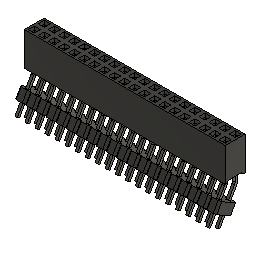
4862 CyberDeck Bonnet (Autodesk Fusion 360 archive; units mm, degrees)
design "2x20 Header 150 degree"
Autodesk Fusion 360 part; units mm, degrees
sketch "Sketch1" plane through (0, 0, 0) normal (1, 0, 0) x (0, 1, 0) in component "header"
  line L0 (-2, 0) -> (-1.7113, 0.5)
  line L1 (-1.7113, 0.5) -> (1.7113, 0.5)
  line L2 (1.7113, 0.5) -> (2, 0)
  line L3 (2, 0) -> (2.5, 0)
  line L4 (2.5, 0) -> (2.5, 8.5)
  line L5 (2.5, 8.5) -> (-2.5, 8.5)
  line L6 (-2.5, 8.5) -> (-2.5, 0)
  line L7 (-2.5, 0) -> (-2, 0)
  line L8 (0, 0.5) -> (0, 0) construction
  line L9 (0, 0.5) -> (0, 8.5) construction
  line L10 (1.27, 0.5) -> (1.27, -2.06)
  line L11 (1.27, -2.06) -> (-3.23, -9.8542)
  line L12 (-1.27, 0.5) -> (-1.27, -1)
  line L13 (-1.27, -1) -> (-5.594, -8.4894)
  line L14 (-5.594, -8.4894) -> (-3.23, -9.8542) construction
  line L15 (-5.0771, -5.3237) -> (-0.7469, -7.8237)
  line L16 (-0.7469, -7.8237) -> (0.5231, -5.624)
  line L17 (0.5231, -5.624) -> (-3.8071, -3.124)
  line L18 (-3.8071, -3.124) -> (-5.0771, -5.3237)
  line L19 (-2.912, -6.5737) -> (-4.412, -9.1718) construction
  dimension "d1" = 5
  dimension "d2" = 8.5
  dimension "d3" = 0.5
  dimension "d4" = 0.5
  dimension "d5" = 0.5
  dimension "d6" = 120
  dimension "d7" = 0.5
  dimension "d8" = 2.56
  dimension "d9" = 9
  dimension "d10" = 1.27
  dimension "d11" = 1.5
  dimension "d12" = 1.27
  dimension "d13" = 150
  dimension "d14" = 2.54
  dimension "d15" = 3
  dimension "d16" = 5
  constraint horizontal L1
  constraint parallel L1 L3
  constraint perpendicular L3 L4
  constraint perpendicular L4 L5
  constraint perpendicular L5 L6
  constraint perpendicular L6 L7
  constraint midpoint L1 L8.start
  constraint coincident L8.end origin
  constraint vertical L8
  constraint midpoint L5 L9.end
  constraint vertical L9
  constraint collinear L3 L7
  constraint coincident L1 L10.start
  constraint perpendicular L1 L10
  constraint coincident L1 L12.start
  constraint perpendicular L1 L12
  constraint parallel L11 L13
  constraint perpendicular L13 L14
  constraint coincident L11.end L14.end
  constraint perpendicular L11 L15
  constraint perpendicular L15 L16
  constraint perpendicular L17 L18
  constraint perpendicular L16 L17
  constraint coincident L15.start L18.end
  constraint midpoint L15 L19.start
  constraint midpoint L14 L19.end
  constraint perpendicular L15 L19
  measures "d1" distance of L4.end L5.end
  measures "d2" distance of L8.end L5
  measures "d3" distance of L2.end L3.end
  measures "d4" distance of L0.start L6.end
  measures "d5" distance of L1 L7
  measures "d6" angle of L0 L7
  measures "d7" distance of L8.start L8.end
  measures "d8" distance of L10.start L10.end
  measures "d9" distance of L10.end L11.end
  measures "d10" distance of L8.end L10
  measures "d11" distance of L12.start L12.end
  measures "d12" distance of L9 L12
  measures "d13" angle of L12 L13
  measures "d14" distance of L17.end L15.start
  measures "d15" distance of L19.start L19.end
  measures "d16" distance of L16.end L17.end
sketch "Sketch2" plane through (0, 0, 0) normal (0, 0, 1) x (1, 0, 0) in component "header"
  line L0 (0.95, 1.59) -> (1.59, 1.59)
  line L1 (1.59, 1.59) -> (1.59, 0.95)
  line L2 (1.59, 0.95) -> (0.95, 0.95)
  line L3 (0.95, 0.95) -> (0.95, 1.59)
  line L4 (1.27, 1.59) -> (1.27, 1.27) construction
  line L5 (1.27, 1.27) -> (1.59, 1.27) construction
  line L6 (0, 0) -> (3, 0) construction
  line L7 (0.95, -1.59) -> (1.59, -1.59)
  line L8 (1.59, -1.59) -> (1.59, -0.95)
  line L9 (1.59, -0.95) -> (0.95, -0.95)
  line L10 (0.95, -0.95) -> (0.95, -1.59)
  dimension "d19" = 0.64
  dimension "d20" = 0.64
  dimension "d21" = 1.27
  dimension "d22" = 1.27
  dimension "d45" = 3
  constraint horizontal L0
  constraint vertical L1
  constraint horizontal L2
  constraint vertical L3
  constraint midpoint L0 L4.start
  constraint perpendicular L0 L4
  constraint perpendicular L4 L5
  constraint midpoint L1 L5.end
  constraint coincident L6.start origin
  constraint horizontal L6
  constraint symmetric L0.start L6 L7.start
  constraint symmetric L0.end L6 L7.end
  constraint symmetric L1.end L6 L8.end
  constraint symmetric L2.end L6 L9.end
  measures "d19" distance of L0.start L0.end
  measures "d20" distance of L0.start L2.end
  measures "d21" distance of L5 L6.start
  measures "d22" distance of L6.start L4
  measures "d45" distance of L6.start L6.end
extrude "Extrude1" add sketch "Sketch1" along normal blind 50.8 contours L0 L1 L2 L3 L4 L5 L6 L7 makes body 1 in component "Header Female"
sweep "Sweep1" add profiles "Sketch2" path "Sketch1" along L10 L11 section 1 contours L0 L1 L2 L3 separate body makes body 2 in component "Pins"
fillet "Fillet1" radius 1 1 edges at (1.27, 0.95, -1.9743) on bodies 2 in component "Pins"
fillet "Fillet1" radius 1.5 1 edges at (1.27, 1.59, -2.1457) on bodies 2 in component "Pins"
pattern_linear "R-Pattern1" count 20 spacing 2.54 along (1, 0, 0) of bodies 2 makes body 3 at (3.49, -0.2493, -4.9048) makes body 4 at (6.03, -0.2493, -4.9048) makes body 5 at (8.57, -0.2493, -4.9048) makes body 6 at (11.11, -0.2493, -4.9048) makes body 7 at (13.65, -0.2493, -4.9048) makes body 8 at (16.19, -0.2493, -4.9048) makes body 9 at (18.73, -0.2493, -4.9048) makes body 10 at (21.27, -0.2493, -4.9048) makes body 11 at (23.81, -0.2493, -4.9048) makes body 12 at (26.35, -0.2493, -4.9048) makes body 13 at (28.89, -0.2493, -4.9048) makes body 14 at (31.43, -0.2493, -4.9048) makes body 15 at (33.97, -0.2493, -4.9048) makes body 16 at (36.51, -0.2493, -4.9048) makes body 17 at (39.05, -0.2493, -4.9048) makes body 18 at (41.59, -0.2493, -4.9048) makes body 19 at (44.13, -0.2493, -4.9048) makes body 20 at (46.67, -0.2493, -4.9048) makes body 21 at (49.21, -0.2493, -4.9048) in component "Pins"
sweep "Sweep2" add profiles "Sketch2" path "Sketch1" along L12 L13 section 1 contours L7 L8 L9 L10 separate body makes body 22 in component "Pins"
fillet "Fillet2" radius 1 1 edges at (1.27, -1.59, -0.9143) on bodies 22 in component "Pins"
fillet "Fillet2" radius 1.5 1 edges at (1.27, -0.95, -1.0857) on bodies 22 in component "Pins"
pattern_linear "R-Pattern2" count 20 spacing 2.54 along (1, 0, 0) of bodies 22 makes body 23 at (3.49, -2.7306, -3.7432) makes body 24 at (6.03, -2.7306, -3.7432) makes body 25 at (8.57, -2.7306, -3.7432) makes body 26 at (11.11, -2.7306, -3.7432) makes body 27 at (13.65, -2.7306, -3.7432) makes body 28 at (16.19, -2.7306, -3.7432) makes body 29 at (18.73, -2.7306, -3.7432) makes body 30 at (21.27, -2.7306, -3.7432) makes body 31 at (23.81, -2.7306, -3.7432) makes body 32 at (26.35, -2.7306, -3.7432) makes body 33 at (28.89, -2.7306, -3.7432) makes body 34 at (31.43, -2.7306, -3.7432) makes body 35 at (33.97, -2.7306, -3.7432) makes body 36 at (36.51, -2.7306, -3.7432) makes body 37 at (39.05, -2.7306, -3.7432) makes body 38 at (41.59, -2.7306, -3.7432) makes body 39 at (44.13, -2.7306, -3.7432) makes body 40 at (46.67, -2.7306, -3.7432) makes body 41 at (49.21, -2.7306, -3.7432) in component "Pins"
extrude "Extrude2" cut sketch "Sketch2" against normal blind 2.54 from surface at 8.5 bodies 1 in component "Header Female"
chamfer "Chamfer2" distance 0.448 angle 45 8 edges at (1.27, -0.95, 8.5) (0.95, -1.27, 8.5) (1.27, -1.59, 8.5) (1.59, -1.27, 8.5) (0.95, 1.27, 8.5) (1.27, 0.95, 8.5) (1.27, 1.59, 8.5) (1.59, 1.27, 8.5) on bodies 1 in component "Header Female"
pattern_linear "R-Pattern1'" count 20 spacing 2.54 along (1, 0, 0) of "Extrude2", "Chamfer2" in component "Header Female"
extrude "Extrude1'" add sketch "Sketch1" along normal blind 2.54 separate body contours L11 L13 L15 L17 | L13 L15 L17 L18 | L11 L15 L16 L17 makes body 42 in component "Strip"
chamfer "Chamfer1" distance 0.5 angle 45 4 edges at (2.54, -4.4421, -4.2239) (2.54, -0.1119, -6.7239) (0, -0.1119, -6.7239) (0, -4.4421, -4.2239) on bodies 42 in component "Strip"
sketch "Sketch1 (2)" plane through (0, -2.3045, -3.9915) normal (0, 0.5, 0.866025) x (-1, 0, 0) in component "Strip"
  line L0 (-1.59, -1.8099) -> (-0.95, -1.8099)
  line L1 (-0.95, -1.8099) -> (-0.95, -2.4499)
  line L2 (-0.95, -2.4499) -> (-1.59, -2.4499)
  line L3 (-1.59, -2.4499) -> (-1.59, -1.8099)
  line L4 (-0.95, 0.9199) -> (-0.95, 0.2799)
  line L5 (-0.95, 0.2799) -> (-1.59, 0.2799)
  line L6 (-1.59, 0.2799) -> (-1.59, 0.9199)
  line L7 (-1.59, 0.9199) -> (-0.95, 0.9199)
extrude "Extrude2'" cut sketch "Sketch1 (2)" against normal up to surface (2.54 mm away) bodies 42 in component "Strip"
pattern_linear "R-Pattern2'" count 20 spacing 2.54 along (1, 0, 0) of bodies 42 makes body 43 at (4.7633, -3.2136, -6.3996) makes body 44 at (7.3033, -3.2136, -6.3996) makes body 45 at (7.9367, -3.2136, -6.3996) makes body 46 at (12.3833, -3.2136, -6.3996) makes body 47 at (14.9233, -3.2136, -6.3996) makes body 48 at (17.4633, -3.2136, -6.3996) makes body 49 at (20.0033, -3.2136, -6.3996) makes body 50 at (22.5433, -3.2136, -6.3996) makes body 51 at (25.0833, -3.2136, -6.3996) makes body 52 at (27.6233, -3.2136, -6.3996) makes body 53 at (30.1633, -3.2136, -6.3996) makes body 54 at (32.7033, -3.2136, -6.3996) makes body 55 at (33.3367, -3.2136, -6.3996) makes body 56 at (35.8767, -3.2136, -6.3996) makes body 57 at (38.4167, -3.2136, -6.3996) makes body 58 at (40.9567, -3.2136, -6.3996) makes body 59 at (43.4967, -3.2136, -6.3996) makes body 60 at (46.0367, -3.2136, -6.3996) makes body 61 at (48.5767, -3.2136, -6.3996) in component "Strip"
combine "Combine1" operation add target body 42 tool bodies 55 60 61 59 58 56 57 51 52 53 54 50 47 48 49 46 44 45 43 in component "Strip"
component "header" placed x (1, 0, 0) y (0, 1, 0) z (0, 0, 1) at (0, 0, 0)
component "Header Female" placed x (1, 0, 0) y (0, 1, 0) z (0, 0, 1) at (0, 0, 0) in component "header"
component "Pins" placed x (1, 0, 0) y (0, 1, 0) z (0, 0, 1) at (0, 0, 0) in component "header"
component "Strip" placed x (1, 0, 0) y (0, 1, 0) z (0, 0, 1) at (0, 0, 0) in component "header"
equation "d10 = ( 2.54 / 2 ) * 1 mm"
equation "d12 = ( 2.54 / 2 ) * 1 mm"
equation "d21 = ( 2.54 / 2 ) * 1 mm"
equation "d22 = ( 2.54 / 2 ) * 1 mm"
equation "d33 = ( 2.54 * 20 ) * 1 mm"
